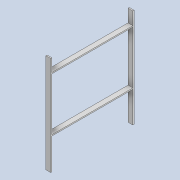
# Autodesk Inventor part: Soporte_molde
Saved by Autodesk Inventor 2021 (Build 250183000, 183)
## iProperties
Created: 2021-04-16
Part Number: Soporte_molde
Material: Genérico
Document SubType Name: Modeling
Designer: Admin
Density: 1 g/cm^3
Appearance: Valor por defecto
Author: Admin
Autodesk Inventor part; units mm, degrees
ref_plane "YZ Plane" through (0, 0, 0) normal (1, 0, 0) x (0, 1, 0)
ref_plane "XZ Plane" through (0, 0, 0) normal (0, 1, 0) x (-1, 0, 0)
ref_plane "XY Plane" through (0, 0, 0) normal (0, 0, 1) x (1, 0, 0)
sketch "Boceto1" plane through (0, 0, 0) normal (1, 0, 0) x (0, 1, 0)
  line L0 (0, 0) -> (-525, 0)
  line L1 (-525, 0) -> (-525, -6.4)
  line L2 (-525, -6.4) -> (0, -6.4)
  line L3 (0, -6.4) -> (0, 0)
  line L4 (-525, -6.4) -> (-354, -6.4)
  line L5 (-354, -6.4) -> (-354, -7.7448)
  line L6 (-354, -6.4) -> (-354, -437.06)
  line L7 (-354, -6.4) -> (-360.4, -6.4)
  line L8 (-360.4, -6.4) -> (-360.4, -437.06)
  line L9 (0, -443.46) -> (-525, -443.46)
  line L10 (-525, -443.46) -> (-525, -437.06)
  line L11 (-525, -437.06) -> (0, -437.06)
  line L12 (0, -437.06) -> (0, -443.46)
  line L13 (-354, -437.06) -> (-74, -437.06)
  line L14 (-74, -437.06) -> (-74, -6.4)
  line L15 (-74, -437.06) -> (-67.6, -437.06)
  line L16 (-67.6, -437.06) -> (-67.6, -6.4)
  dimension "d0" = 525
  dimension "d1" = 6.4
  dimension "d2" = 171
  dimension "d3" = 430.66
  dimension "d4" = 6.4
  dimension "d5" = 430.66
  dimension "d6" = 280
  dimension "d7" = 6.4
  constraints: 34 end point, 6 perpendicular, 6 point on line, 2 vertical, 1 horizontal
  measures "d0" distance of L0.start L0.end
  measures "d1" distance of L0.end L1.end
  measures "d2" distance of L1.end L4.end
  measures "d3" distance of L4.end L6.end
  measures "d4" distance of L4.end L7.end
  measures "d5" distance of L7.end L8.end
  measures "d6" distance of L6.end L13.end
  measures "d7" distance of L13.end L15.end
extrude "Extrusión1" add sketch "Boceto1" along normal blind 25.4 contours L3 L2 L1 L0 | L16 L11 L14 L2 | L2 L5 L6 L11 L8 | L11 L12 L9 L10
